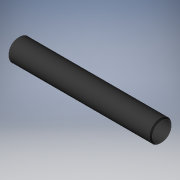
# Autodesk Inventor part: 0.75-5.303x0.810_body
Saved by Autodesk Inventor 2019 (Build 230136000, 136)
## iProperties
Created: 2023-02-15
Part Number: 0.75-5.303x0.810_body
Material: Generic
Catalog Web Link: www.cadenas.de
Description: SR Series Body-Pneumatic Cylinder
Vendor: PARKERHANNIFIN
Document SubType Name: Modeling
Designer: psAdmin
Manufacturer: PARKERHANNIFIN
Mass: 5.55462 g
Surface Area: 169.337 cm^2
Volume: 5.55462 cm^3
Density: 1 g/cm^3
Appearance: PSOLRGB-175-175-175
Category: PARTsolutions
Company: PARKERHANNIFIN
Title: 0.75-5.303x0.810_body
Author: Cadenas PARTsolutions
Comments: Pneumatic Cylinder
PSOL_IDENT_0: {$CADENAS_DATA/23d-libs/parkerpdn/actuators_cylinders/pneumatic_cylinders/sr_series/parts/sr_body.pr
PSOL_IDENT_1: j},200 {VTYP=3D},{NB=0.75-5.303x0.810_body},{LINA=0.75-5.303x0.810_body},{NN=SR Series Body},{DATE=2
PSOL_IDENT_2: 6.07.2021 05:25:39},{GEOMDATE=23.03.2020 15:15:49},{VERSION=},{LINEID=40},{WBVAR=L,X2D},{WBNUMERIC=L
PSOL_IDENT_3: ,X2D}  {NB=0.75-5.303x0.810_body},{LINA=0.75-5.303x0.810_body},{KT=DUMMY},{PN=0.75-5.303x0.810_body}
PSOL_IDENT_4: ,{BORE=0.7500},{BORECON=0.7500},{L=5.30300},{OD=0.81000},{D1=0.70100},{D2=0.75800},{C1=0.03000},{L4=
PSOL_IDENT_5: 0.03600},{X2D=0}
NB: 0.75-5.303x0.810_body
NN: SR Series Body
NT: Pneumatic Cylinder
NBSYN: $PN.
LINA: 0.75-5.303x0.810_body
CATALOG: Parker Pneumatic Division
BORE: 0.75
BORECON: 0.7500
L: 5.303
OD: 0.81
D1: 0.701
D2: 0.758
C1: 0.03
L4: 0.036
X2D: 0
SUPPLIER: PARKERHANNIFIN
ARTICLENO: 0.75-5.303x0.810_body
BOMINFO: 0.75-5.303x0.810_body
CREATOR: CADENAS GmbH
Autodesk Inventor part; units mm, degrees
sketch "Sketch_1" plane through (0, 0, 0) normal (0, 0, 1) x (1, 0, 0)
  line L0 (67.3481, 0) -> (-67.3481, 0)
  line L1 (-67.3481, 8.9027) -> (-66.4337, 8.9027)
  line L2 (-66.4337, 8.9027) -> (-65.7098, 9.6266)
  line L3 (-65.7098, 9.6266) -> (65.7098, 9.6266)
  line L4 (65.7098, 9.6266) -> (66.4337, 8.9027)
  line L5 (66.4337, 8.9027) -> (67.3481, 8.9027)
  line L6 (67.3481, 8.9027) -> (65.9638, 10.287)
  line L7 (65.9638, 10.287) -> (-65.9638, 10.287)
  line L8 (-65.9638, 10.287) -> (-67.3481, 8.9027)
  constraints: 18 end point
revolve "Revolution1" add sketch "Sketch_1" angle 360 about axis through (67.3481, 0, 0) along (1, 0, 0)
ref_plane "cap_XY" through (67.3481, 0, 0) normal (1, 0, 0) x (0, 0, -1)
ref_plane "cap_YZ" through (67.3481, 0, 0) normal (0, 0, -1) x (0, 1, 0)
ref_plane "cap_ZX" through (67.3481, 0, 0) normal (0, 1, 0) x (1, 0, 0)
ref_plane "head_XY" through (-67.3481, 0, 0) normal (1, 0, 0) x (0, 0, -1)
ref_plane "head_YZ" through (-67.3481, 0, 0) normal (0, 0, -1) x (0, 1, 0)
ref_plane "head_ZX" through (-67.3481, 0, 0) normal (0, 1, 0) x (1, 0, 0)
body "Solid1"
